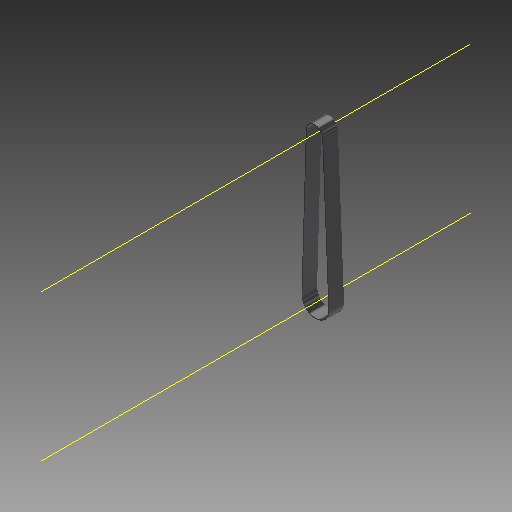
# Autodesk Inventor part: Zahnriemen
Saved by Autodesk Inventor 2019 (Build 230136000, 136)
## iProperties
Created: 2021-04-25
Part Number: Zahnriemen
Material: Rubber
Document SubType Name: Modeling
Designer: Michael Sumper
Density: 1 g/cm^3
Appearance: Rubber - Black - Version 1.1
CustomPartVersion: 1
Author: Michael Sumper
Autodesk Inventor part; units mm, degrees
sketch "Skizzenpfad" plane through (0, 0, 0) normal (0, 0, 1) x (1, 0, 0)
  arc A0 (5.5654, 0.2358) -> (-5.5679, 0.1674) centre (0, 0) ccw
  arc A1 (-8.5391, -98.6742) -> (9.7513, -98.5618) centre (0.6081, -98.9492) ccw
  line L0 (-8.5391, -98.6742) -> (-5.5679, 0.1674)
  line L1 (5.5654, 0.2358) -> (9.7513, -98.5618)
  constraints: 4 end point, 2 point on circle, 1 centre point, 3 other
ref_plane "Querschnittsebene" through (-5.5679, 0.1674, 0) normal (-0.03, -0.9995, 0) x (0, 0, 1)
ref_plane "Arbeitsebene2" through (0, 0, 0) normal (-1, 0, 0) x (0, 0, 1)
ref_plane "Arbeitsebene3" through (0.6081, -98.9492, 0) normal (-0.0315, 0.9995, 0) x (0, 0, 1)
sketch "Querschnitt" plane through (-5.5679, 0.1674, 0) normal (-0.03, -0.9995, 0) x (0, 0, 1)
  line L0 (-5, 0.3) -> (5, 0.3)
  line L1 (5, 0.3) -> (5, -0.3)
  line L2 (5, -0.3) -> (-5, -0.3)
  line L3 (-5, -0.3) -> (-5, 0.3)
  line L4 (-5, 0) -> (5, 0) construction
  point P0 (0, 0)
  point P1 (0, 0)
  dimension "d0" = 10
  dimension "d4" = 0.3
  dimension "d5" = 0.3
  constraints: 10 end point, 3 midpoint, 2 parallel, 1 coincident, 1 horizontal, 1 perpendicular, 1 other
  measures "d0" distance between parallel lines of L1 L3
  measures "d4" distance between parallel lines of L2 L4
  measures "d5" distance between parallel lines of L4 L0
sweep "Riemen" add profiles "Querschnitt" path "Skizzenpfad"
equation "\"d0\" = da_B"
equation "\"d4\" = da_a"
equation "\"d5\" = da_a2"
equation "\"da_B\" = 10"
equation "\"da_pb\" = 2.5"
equation "\"da_L\" = 244.28178"
equation "\"da_a\" = 0.3"
equation "\"da_S\" = 1.5"
equation "\"da_Beta\" = 20deg"
equation "\"da_Ht\" = 0.7"
equation "\"da_H\" = 1.3"
equation "\"da_a2\" = 0.3"
body "Solid1"
